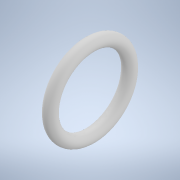
# Autodesk Inventor part: silicon-ring-mockup
Saved by Autodesk Inventor 2021 (Build 250183000, 183)
## iProperties
Created: 2024-05-06
Part Number: silicon-ring-mockup
Material: Generic
Document SubType Name: Modeling
Designer: Toby
Density: 1 g/cm^3
Appearance: Default
Author: Toby
Autodesk Inventor part; units mm, degrees
ref_plane "YZ Plane" through (0, 0, 0) normal (1, 0, 0) x (0, 1, 0)
ref_plane "XZ Plane" through (0, 0, 0) normal (0, 1, 0) x (-1, 0, 0)
ref_plane "XY Plane" through (0, 0, 0) normal (0, 0, 1) x (1, 0, 0)
sketch "Sketch1" plane through (0, 0, 0) normal (0, 0, 1) x (1, 0, 0)
  circle A0 centre (0, 16.5) radius 2.5
  line L0 (-3.5, 0) -> (3.5, 0) projected
  point P0 (0, 0)
  point P1 (2.2913, 0)
  point P2 (-2.2913, 0)
  dimension "d0" = 5
  dimension "d1" = 16.5
  constraints: 1 centre point
  measures "d0" diameter of A0
  measures "d1" distance of point (0, 0) A0.centre
revolve "Revolution1" add sketch "Sketch1" angle 360 about axis through (-10, 0, 0) along (1, 0, 0)
body "Solid1"
